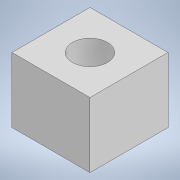
# Autodesk Inventor part: sliding_lifter
Saved by Autodesk Inventor 2022 (Build 260153000, 153)
## iProperties
Created: 2021-07-08
Part Number: sliding_lifter
Material: Generic
Document SubType Name: Modeling
Designer: fraaw
Density: 1 g/cm^3
Appearance: Default
Author: fraaw
## iProperties of the stored document sliding_lifter_3DPrint.ipt
Created: 2021-07-08
Part Number: sliding_lifter_3DPrint
Material: Generic
Document SubType Name: Modeling
Designer: fraaw
Density: 1 g/cm^3
Appearance: Default
Author: fraaw
Autodesk Inventor part; units mm, degrees
ref_plane "YZ Plane" through (0, 0, 0) normal (1, 0, 0) x (0, 1, 0)
ref_plane "XZ Plane" through (0, 0, 0) normal (0, 1, 0) x (-1, 0, 0)
ref_plane "XY Plane" through (0, 0, 0) normal (0, 0, 1) x (1, 0, 0)
sketch "Sketch1" plane through (0, 0, 0) normal (0, 1, 0) x (-1, 0, 0)
  line L0 (-9.6, 9.6) -> (9.6, 9.6)
  line L1 (9.6, 9.6) -> (9.6, -9.6)
  line L2 (9.6, -9.6) -> (-9.6, -9.6)
  line L3 (-9.6, -9.6) -> (-9.6, 9.6)
  line L4 (-9.6, 9.6) -> (9.6, -9.6) construction
  line L5 (9.6, 9.6) -> (-9.6, -9.6) construction
  circle A0 centre (0, 0) radius 4.3
  dimension "d0" = 19.2
  dimension "d1" = 19.2
  dimension "d2" = 8.6
  constraints: 12 end point, 2 midpoint, 2 parallel, 1 centre point, 1 coincident, 1 horizontal, 1 perpendicular
  measures "d0" distance of L0.end L1.end
  measures "d1" distance of L1.end L2.end
  measures "d2" diameter of A0
extrude "Extrusion1" add sketch "Sketch1" along normal blind 16
body "Solid1"
